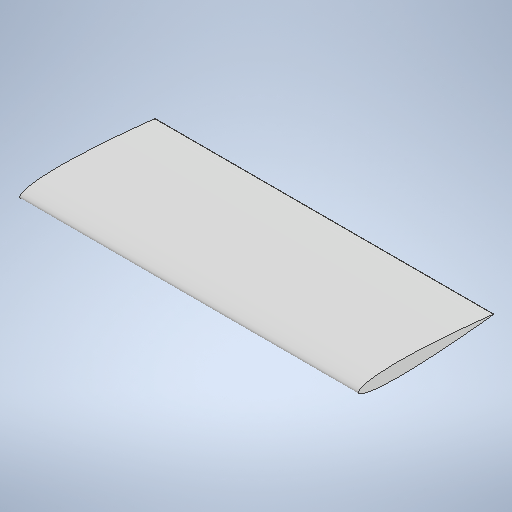
# Autodesk Inventor part: Wing_horizontal
Saved by Autodesk Inventor 2027.1 (Build 311270010, 270A)
## iProperties
Created: 2026-09-09
Part Number: Wing_horizontal
Material: Generic
Document SubType Name: Modeling
Designer: PWYNNE
Density: 1 g/cm^3
Appearance: Default
Author: PWYNNE
Autodesk Inventor part; units mm, degrees
ref_plane "YZ Plane" through (0, 0, 0) normal (1, 0, 0) x (0, 1, 0)
ref_plane "XZ Plane" through (0, 0, 0) normal (0, 1, 0) x (-1, 0, 0)
sketch "Sketch1" plane through (0, 0, 0) normal (1, 0, 0) x (0, 1, 0)
  spline S0 degree 4 poles (0.1575, -150) (0.9442, -143.0257) (1.2416, -140.7856) (3.1541, -122.1812) (4.6023, -104.9702) (5.761, -90.0485) (6.6458, -74.9345) (7.3031, -62.0682) (7.5406, -45.612) (7.4957, -38.7178) (7.2162, -30.0309) (6.8321, -23.4884) (5.9983, -15.3873) (5.3066, -11.6853) (4.7384, -8.0548) (3.1787, -3.5028) (2.8427, -2.3681) (0, 1.5418) (-2.8427, -2.3681) (-3.1787, -3.5028) (-4.7384, -8.0548) (-5.3066, -11.6853) (-5.9984, -15.3873) (-6.8318, -23.4884) (-7.2175, -30.0309) (-7.4916, -38.7178) (-7.5548, -45.612) (-7.2965, -62.0681) (-6.6484, -74.9345) (-5.7601, -90.0484) (-4.6026, -104.9702) (-3.1539, -122.1812) (-1.2417, -140.7856) (-0.9442, -143.0257) (-0.1575, -150) knots 0 0 0 0 0 0.079089 0.115945 0.155696 0.195428 0.235142 0.271937 0.305818 0.336796 0.364889 0.390959 0.415029 0.437154 0.455937 0.474178 0.491854 0.508146 0.525822 0.544063 0.562846 0.584971 0.60904 0.63511 0.663203 0.694182 0.728063 0.764858 0.804572 0.844304 0.884055 0.920911 1 1 1 1 1
  line L0 (0.1575, -150) -> (-0.1575, -150)
  line L1 (0, 0) -> (0, -150) construction
  line L2 (7.497, -90) -> (7.497, 0) construction
  line L3 (-7.503, -90) -> (-7.503, 0) construction
  point P0 (1.008, -142.5)
  point P1 (1.8105, -135)
  point P2 (3.2805, -120)
  point P3 (4.5795, -105)
  point P4 (5.7045, -90)
  point P5 (6.618, -75)
  point P6 (7.2555, -60)
  point P7 (7.497, -45)
  point P8 (7.428, -37.5)
  point P9 (7.173, -30)
  point P10 (6.6825, -22.5)
  point P11 (5.853, -15)
  point P12 (5.25, -11.25)
  point P13 (4.443, -7.5)
  point P14 (3.267, -3.75)
  point P15 (2.367, -1.875)
  point P16 (-2.367, -1.875)
  point P17 (-3.267, -3.75)
  point P18 (-4.443, -7.5)
  point P19 (-5.25, -11.25)
  point P20 (-5.853, -15)
  point P21 (-6.6825, -22.5)
  point P22 (-7.173, -30)
  point P23 (-7.428, -37.5)
  point P24 (-7.503, -45)
  point P25 (-7.2555, -60)
  point P26 (-6.618, -75)
  point P27 (-5.7045, -90)
  point P28 (-4.5795, -105)
  point P29 (-3.2805, -120)
  point P30 (-1.8105, -135)
  point P31 (-1.008, -142.5)
  point P32 (0, -75)
  point P33 (0, -37.5)
  dimension "d1" = 150
  dimension "d2" = 75
  dimension "d3" = 37.5
  dimension "d5" = 15
  constraints: 8 end point, 4 midpoint, 1 horizontal, 1 parallel, 1 point on line, 1 vertical, 35 other
  measures "d1" distance of L1.start L1.end
  measures "d2" distance of point (0, 0) point (0, -75)
  measures "d3" distance of point (0, 0) point (0, -37.5)
  measures "d5" distance between parallel lines of L3 L2
ref_plane "Work Plane1" through (0, 0, -37.5) normal (0, 0, 1) x (1, 0, 0)
extrude "Extrusion1" add sketch "Sketch1" along normal blind 375
body "Solid1"
